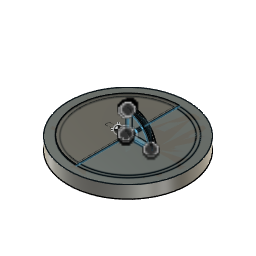
Automatic trash bin v3 (Autodesk Fusion 360 design; units mm, degrees)
Autodesk Fusion 360 part; units mm, degrees
sketch "Sketch1" plane through (0, 0, 0) normal (0, 0, 1) x (1, 0, 0)
  circle A0 centre (175, 175) radius 142.5
  circle A1 centre (175, 175) radius 132.5
  dimension "d2" = 285
  dimension "d3" = 265
  constraint concentric A0 A1
  measures "d2" diameter of A0
  measures "d3" diameter of A1
extrude "Extrude1" add sketch "Sketch1" along normal blind 20 makes body 1
sketch "Sketch2" plane through (0, 0, 20) normal (0, 0, 1) x (-1, 0, 0)
  circle A0 centre (-175, -175) radius 132.5
  circle A1 centre (-175, -175) radius 142.5
extrude "Extrude2" add sketch "Sketch2" along normal blind 10 contours A0 | A1 bodies 1
sketch "Sketch3" plane through (0, 0, 30) normal (0, 0, 1) x (-1, 0, 0)
  circle A0 centre (-175, -175) radius 142.5
  circle A1 centre (-175, -175) radius 122.5
  circle A2 centre (-175, -175) radius 115
  line L0 (-175, -175) -> (-175, -170)
  line L1 (-175, -175) -> (-175, -180)
  line L2 (-175, -170) -> (-235, -170)
  line L3 (-175, -180) -> (-235, -180)
  line L4 (-175, -180) -> (-175, -290)
  line L5 (-175, -170) -> (-175, -60)
  line L6 (-235, -180) -> (-235, -170)
  line L7 (-175, -290) -> (-175, -297.5)
  line L8 (-175, -60) -> (-175, -52.5)
  dimension "d8" = 245
  dimension "d9" = 230
  dimension "d15" = 5
  dimension "d16" = 5
  dimension "d17" = 60
  constraint concentric A0 A1
  constraint concentric A1 A2
  constraint coincident A0.centre A1.centre
  constraint perpendicular L0 L2
  constraint perpendicular L1 L3
  constraint coincident A2 L4.end
  constraint perpendicular L3 L4
  constraint coincident A2 L5.end
  constraint perpendicular L2 L5
  constraint perpendicular L2 L6
  constraint coincident A1 L7.end
  constraint parallel L4 L7
  constraint coincident A1 L8.end
  constraint parallel L5 L8
  measures "d8" diameter of A1
  measures "d9" diameter of A2
  measures "d15" distance of A0.centre L0.end
  measures "d16" distance of A0.centre L1.end
  measures "d17" distance of L0.end L2.end
extrude "Extrude4" cut sketch "Sketch3" against normal blind 10 contours A2 L0 L1 L4 L5 bodies 1
extrude "Extrude5" add sketch "Sketch3" along normal blind 60 separate body contours L0 L1 L2 L3 L6 makes body 2
sketch "Sketch4" plane through (0, 170, 0) normal (0, -1, 0) x (1, 0, 0)
  line L0 (175, 30) -> (235, 30)
  line L1 (235, 30) -> (235, 90)
  line L2 (235, 90) -> (175, 90)
  line L3 (175, 90) -> (175, 30)
  line L4 (175, 30) -> (235, 30)
  arc A0 (235, 30) -> (175, 90) centre (175, 30) ccw
  arc A1 (230, 30) -> (175, 85) centre (175, 30) ccw
  arc A2 (185, 30) -> (175, 40) centre (175, 30) ccw
  line L5 (180, 90) -> (180, 30)
  line L6 (235, 35) -> (175, 35)
  line L7 (217.4264, 72.4264) -> (175, 30)
  line L8 (200, 55) -> (201.7678, 53.2322)
  line L9 (200, 55) -> (198.2322, 56.7678)
  line L10 (198.2322, 56.7678) -> (215.6218, 74.1573)
  line L11 (201.7678, 53.2322) -> (219.1573, 70.6218)
  line L12 (201.7678, 53.2322) -> (178.5355, 30)
  line L13 (198.2322, 56.7678) -> (175, 33.5355)
  dimension "d41" = 2.5
  dimension "d42" = 2.5
  constraint coincident L0.end L1.start
  constraint coincident L0.start L3.end
  constraint coincident L2.end L3.start
  constraint coincident L3 A1.end
  constraint coincident L4 A1.start
  constraint coincident L3 A2.end
  constraint coincident L4 A2.start
  constraint coincident L2 L5.start
  constraint coincident L4 L5.end
  constraint perpendicular L4 L5
  constraint coincident L1 L6.start
  constraint coincident L3 L6.end
  constraint perpendicular L3 L6
  constraint midpoint A0 L7.start
  constraint coincident L7 L8.start
  constraint perpendicular L7 L8
  constraint perpendicular L7 L9
  constraint coincident A0 L10.end
  constraint perpendicular L9 L10
  constraint coincident A0 L11.end
  constraint perpendicular L8 L11
  constraint coincident L4 L12.end
  constraint perpendicular L8 L12
  constraint coincident L3 L13.end
  constraint perpendicular L9 L13
  measures "d41" distance of L8.start L8.end
  measures "d42" distance of L8.start L9.end
extrude "Extrude7" add sketch "Sketch3" along normal blind 2 separate body contours A1 A2 L7 L8 | A2 L0 L1 L4 L5 picked at (-163.7334, -55.8058) makes body 3
extrude "Extrude8" cut sketch "Sketch3" against normal blind 10 contours L0 L1 L2 L3 L6 bodies 1
extrude "Extrude9" add sketch "Sketch3" against normal blind 30 contours L0 L1 L2 L3 L6 bodies 2
move_face "OffsetFaces1" offset 5 2 faces at (175, 133.3333, 26.6667) (175, 253.3333, 26.6667) on bodies 1
extrude "Extrude11" cut sketch "Sketch4" against normal blind 10 contours A1 A2 L5 L10 L13 | A1 A2 L6 L11 L12 | L1 A0 L6 | L2 A0 L5 | L1 L2 A0 L5 L6 bodies 2
sketch "Sketch5" plane through (175, 0, 0) normal (-1, 0, 0) x (0, -1, 0)
  line L0 (-170, 0) -> (-170, 90)
  line L1 (-170, 90) -> (-180, 90)
  line L2 (-180, 90) -> (-180, 0)
  line L3 (-180, 0) -> (-170, 0)
  line L4 (-170, 30) -> (-180, 30)
  line L5 (-180, 90) -> (-178, 90)
  line L6 (-170, 90) -> (-172, 90)
  line L7 (-178, 90) -> (-177, 88)
  line L8 (-177, 88) -> (-175, 87)
  line L9 (-175, 87) -> (-173, 88)
  line L10 (-173, 88) -> (-172, 90)
  line L11 (-178, 90) -> (-179, 93)
  line L12 (-179, 93) -> (-180, 93)
  line L13 (-180, 93) -> (-180, 90)
  line L14 (-172, 90) -> (-171, 93)
  line L15 (-171, 93) -> (-170, 93)
  line L16 (-170, 93) -> (-170, 90)
  line L17 (-179, 93) -> (-171, 93)
  line L18 (-175, 87) -> (-175, 88.5)
  circle A0 centre (-175, 88.5) radius 0.75
  dimension "d51" = 1.5
  constraint coincident L0 L4.start
  constraint coincident L2 L4.end
  constraint perpendicular L2 L4
  constraint coincident L1.end L2.start
  constraint coincident L1 L5.end
  constraint perpendicular L2 L5
  constraint coincident L0.end L1.start
  constraint coincident L1 L6.end
  constraint perpendicular L0 L6
  constraint parallel L5 L12
  constraint parallel L6 L15
  constraint parallel L15 L17
  constraint vertical L18
  constraint coincident L18.end A0.centre
  measures "d51" diameter of A0
extrude "Extrude12" add sketch "Sketch5" along normal blind 50 contours L0 L2 L3 L4 bodies 2
chamfer "Chamfer2" distance 30 distance2 90 1 edges at (125, 175, 0) measured on face at (125, 173.3333, 10) on bodies 2
revolve "Revolve1" cut sketch "Sketch5" angle 90 about axis through (175, 170, 30) along (0, 1, 0) contours L1 L6 L14 L15 L16 | L1 L7 L8 L9 L10 | L1 L5 L11 L12 L13 | A0 bodies 2
revolve "Revolve2" add sketch "Sketch5" angle 90 about axis through (175, 170, 30) along (0, 1, 0) contours L1 L6 L14 L15 L16 | L1 L5 L11 L12 L13 bodies 2
extrude "Extrude13" add sketch "Sketch5" against normal blind 3 separate body contours L1 L7 L8 L9 L10 | L1 L11 L14 L17 | A0 makes body 4
extrude "Extrude14" cut sketch "Sketch5" against normal blind 3 contours A0 bodies 4
combine "Combine1" operation add target body 2 tool bodies 4
sketch "Sketch6" plane through (0, 0, 30) normal (0, 0, 1) x (-1, 0, 0)
  line L0 (-235, -172) -> (-233, -173)
  line L1 (-233, -173) -> (-232, -175)
  line L2 (-232, -175) -> (-233, -177)
  line L3 (-233, -177) -> (-235, -178)
  line L4 (-235, -178) -> (-235, -172)
  line L5 (-235, -172) -> (-238, -171)
  line L6 (-238, -171) -> (-238, -170)
  line L7 (-238, -170) -> (-235, -170)
  line L8 (-235, -170) -> (-235, -172)
  line L9 (-235, -178) -> (-235, -180)
  line L10 (-235, -180) -> (-238, -180)
  line L11 (-238, -180) -> (-238, -179)
  line L12 (-238, -179) -> (-235, -178)
  constraint vertical L4
  constraint parallel L4 L6
  constraint perpendicular L4 L7
  constraint perpendicular L7 L8
  constraint parallel L4 L9
  constraint perpendicular L4 L10
  constraint perpendicular L10 L11
extrude "Extrude15" cut sketch "Sketch6" against normal blind 30 contours L0 L1 L2 L3 L4 bodies 2
extrude "Extrude16" add sketch "Sketch6" against normal blind 30 contours L9 L10 L11 L12 | L5 L6 L7 L8 bodies 2
combine "Combine2" operation cut target body 1 tool bodies 2 keep tools
